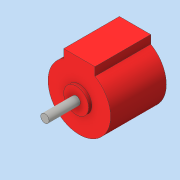
# Autodesk Inventor part: Minebea_SMS6-20_StepperMotor_Mockup
Saved by Autodesk Inventor 2016 (Build 200138000, 138)
## iProperties
Created: 2017-10-09
Part Number: Minebea_SMS6-20_StepperMotor_Mockup
Material: Generic
Document SubType Name: Modeling
Designer: rahul
Density: 1 g/cm^3
Appearance: Default
Author: rahul
Autodesk Inventor part; units mm, degrees
ref_plane "YZ Plane" through (0, 0, 0) normal (1, 0, 0) x (0, 1, 0)
ref_plane "XZ Plane" through (0, 0, 0) normal (0, 1, 0) x (-1, 0, 0)
ref_plane "XY Plane" through (0, 0, 0) normal (0, 0, 1) x (1, 0, 0)
sketch "Sketch1" plane through (0, 0, 0) normal (0, 0, 1) x (1, 0, 0)
  circle A0 centre (0, 0) radius 3
  line L0 (-1.5, 2.5981) -> (-1.5, 3.4)
  line L1 (-1.5, 3.4) -> (1.5, 3.4)
  line L2 (1.5, 3.4) -> (1.5, 2.5981)
  line L3 (0, 4.68) -> (0, -4.28) projected
  line L4 (-4.2, 0) -> (4.2, 0) projected
  dimension "d0" = 6
  dimension "d1" = 3.4
  dimension "d2" = 3
  constraints: 6 end point, 2 perpendicular, 2 point on circle, 1 centre point, 1 coincident, 1 vertical, 1 other
  measures "d0" diameter of A0
  measures "d1" distance between parallel lines of L1 L4
  measures "d2" distance of L0.end L1.end
extrude "Body" add sketch "Sketch1" against normal blind 5.35
sketch "Sketch2" plane through (0, 0, 0) normal (0, 0, 1) x (1, 0, 0)
  circle A0 centre (0, 0) radius 1.2
  dimension "d5" = 2.4
  constraints: 1 centre point, 1 coincident
  measures "d5" diameter of A0
extrude "Face Boss" add sketch "Sketch2" along normal blind 0.3
sketch "Sketch3" plane through (0, 0, 0.3) normal (0, 0, 1) x (1, 0, 0)
  circle A0 centre (0, 0) radius 0.4
  dimension "d8" = 0.8
  constraints: 1 centre point, 1 coincident
  measures "d8" diameter of A0
extrude "Extrusion3" add sketch "Sketch3" along normal blind 3
body "Solid1"
